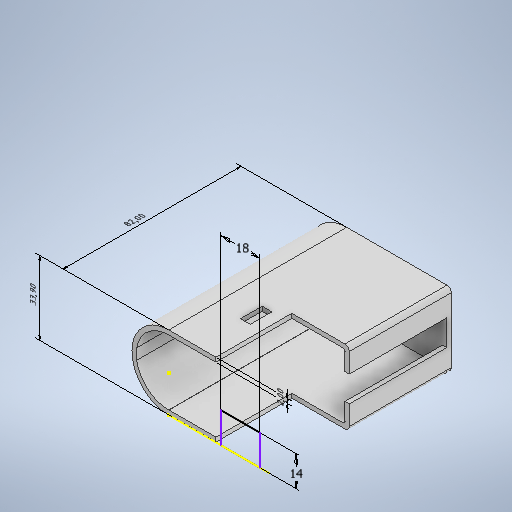
# Autodesk Inventor part: schranka
Saved by Autodesk Inventor 2025.3 (Build 293356000, 356)
## iProperties
Created: 2025-06-12
Part Number: schranka
Material: Generic
Document SubType Name: Modeling
Designer: Repete
Density: 1 g/cm^3
Appearance: Default
Author: Repete
Autodesk Inventor part; units mm, degrees
ref_plane "YZ Plane" through (0, 0, 0) normal (1, 0, 0) x (0, 1, 0)
ref_plane "XZ Plane" through (0, 0, 0) normal (0, 1, 0) x (-1, 0, 0)
sketch "Sketch1" plane through (0, 0, 0) normal (0, 1, 0) x (-1, 0, 0)
  line L0 (-15.6488, -14.9) -> (-4.1777, -14.9)
  line L1 (-4.1777, 15) -> (-13.2013, 15)
  line L2 (14.7902, 2.5) -> (14.8, 2.5)
  line L3 (14.8, 2.5) -> (14.8, -2.5)
  line L4 (14.8, -2.5) -> (14.7902, -2.5)
  arc A0 (0, -15) -> (14.7902, -2.5) centre (0, 0) ccw
  arc A1 (14.7902, 2.5) -> (0, 15) centre (0, 0) ccw
  line L5 (0.0236, 15) -> (0.0236, 15.0064)
  line L6 (0.0236, 15) -> (-4.1777, 15)
  line L7 (-4.1777, 15) -> (-4.1777, 15)
  line L8 (-0.1777, -14.9) -> (-4.1777, -14.9)
  line L9 (-4.1777, -14.9) -> (0, -14.9)
  line L10 (-4.1777, -14.9) -> (-4.1777, -14.9)
  line L11 (-13.2013, 15) -> (-46.2013, 15)
  line L12 (-15.6488, -14.9) -> (-46.2013, -14.9)
  line L13 (-46.2013, -14.9) -> (-46.2013, 15)
  arc A2 (-1.8412, -16.9) -> (0, 17) centre (0, 0) ccw
  line L14 (0, 17) -> (-48.2013, 17)
  line L15 (-48.2013, 17) -> (-48.2013, -16.9)
  line L16 (-48.2013, -16.9) -> (-1.8412, -16.9)
  line L17 (0.0236, 15) -> (0.0236, 15)
  line L18 (0, -14.9) -> (0, -15)
  point P0 (-13.2013, 0)
  point P1 (12.5, 0)
  point P2 (11.0065, 21.7068)
  point P3 (11.0065, 50.7004)
  dimension "d7" = 33
  dimension "d8" = 2
  dimension "d9" = 2
  dimension "d10" = 2
  dimension "d11" = 2
  dimension "d39" = 15
  dimension "d90" = 33.9
  dimension "d91" = 29.9
  dimension "d92" = 2
  dimension "d93" = 2
  dimension "d94" = 2.2
  dimension "d95" = 14.8
  constraints: 38 end point, 7 point on circle, 5 horizontal, 4 parallel, 4 perpendicular, 3 centre point, 1 coincident, 1 vertical
  measures "d7" distance from line of L13 point (-13.201, 0)
  measures "d8" radial gap between concentric circles of A0 A2
  measures "d9" distance between parallel lines of L15 L13
  measures "d10" distance between parallel lines of L0 L16
  measures "d11" distance between parallel lines of L14 L11
  measures "d39" radius of A1
  measures "d90" distance of L14.end L15.end
  measures "d91" distance of L12.end L11.end
  measures "d92" distance between parallel lines of L14 L6
  measures "d93" distance between parallel lines of L16 L8
  measures "d94" distance edge to line of A2 L3
  measures "d95" distance from line of A0.centre L3
extrude "Extrusion1" add sketch "Sketch1" along normal blind 80
ref_plane "Work Plane1" through (0, 82, 0) normal (0, 1, 0) x (1, 0, 0)
sketch "Sketch3" plane through (0, 82, 0) normal (0, 1, 0) x (1, 0, 0)
  arc A0 (0, 17) -> (0, -17) centre (0, 0) ccw
  line L0 (0, -17) -> (48.2013, -17)
  line L1 (48.2013, -17) -> (48.2013, 17)
  line L2 (48.2013, 17) -> (0, 17)
  point P0 (13.2013, 0)
  point P1 (-14.9845, -166.3883)
  point P2 (-14.9845, -137.3947)
  point P3 (-26.1687, -202.0885)
  constraints: 6 end point, 2 point on circle, 1 centre point, 1 parallel, 1 perpendicular
extrude "Extrusion2" add sketch "Sketch3" against normal up to surface (2 mm away)
sketch "Sketch4" plane through (48.2013, 0, -16.9) normal (0, 0, -1) x (-1, 0, 0)
  point P0 (48.2013, 0)
fillet "Fillet1" radius 2 2 edges at (48.2013, 40, -16.9) (48.2013, 41, 17)
fillet "Fillet2" radius 1 2 edges at (46.2013, 40, 15) (46.2013, 40, -14.9)
fillet "Fillet3" radius 2 1 edges at (48.2013, 81, -17)
sketch "Sketch10" plane through (0, 0, 0) normal (0, -1, 0) x (1, 0, 0)
  line L0 (0, -17) -> (46.2013, -17) projected
  line L1 (23.9488, -17) -> (41.9488, -17)
  line L2 (41.9488, -17) -> (41.9488, -3)
  line L3 (41.9488, -3) -> (23.9488, -3)
  line L4 (23.9488, -3) -> (23.9488, -17)
  point P0 (0, 0)
  dimension "d79" = 14
  dimension "d80" = 18
  constraints: 8 end point, 2 parallel, 1 horizontal, 1 perpendicular, 1 point on line
  measures "d79" distance of L1.end L2.end
  measures "d80" distance of L2.end L3.end
sketch "Sketch11" plane through (0, 0, 0) normal (0, -1, 0) x (1, 0, 0)
  line L0 (0, 17) -> (46.2013, 17) projected
  line L1 (21.7013, 17) -> (48.2013, 17)
  line L2 (48.2013, 17) -> (48.2013, -16.9)
  line L3 (48.2013, -16.9) -> (21.7013, -16.9)
  line L4 (21.7013, -16.9) -> (21.7013, 17)
  line L5 (48.2013, 15) -> (48.2013, -14.9) projected
  point P0 (0, 0)
  dimension "d86" = 26.5
  dimension "d87" = 0
  constraints: 8 end point, 2 parallel, 1 horizontal, 1 perpendicular, 1 point on line
  measures "d86" distance between parallel lines of L2 L4
  measures "d87" distance between parallel lines of L5 L2
extrude "Extrusion8" cut sketch "Sketch11" against normal blind 35
sketch "Sketch12" plane through (48.2013, 82, 15) normal (1, 0, 0) x (0, 0, -1)
  line L0 (0, -47) -> (29.9, -47) projected
  line L1 (9, -47) -> (20.9, -47)
  line L2 (20.9, -47) -> (20.9, -2)
  line L3 (20.9, -2) -> (9, -2)
  line L4 (9, -2) -> (9, -47)
  line L5 (29.9, -2) -> (29.9, -47) projected
  line L6 (0, -47) -> (0, 0) projected
  line L7 (0, 0) -> (30, 0) projected
  point P0 (15, -82)
  dimension "d97" = 9
  dimension "d98" = 9
  dimension "d99" = 2
  constraints: 8 end point, 2 parallel, 1 horizontal, 1 perpendicular, 1 point on line
  measures "d97" distance between parallel lines of L5 L2
  measures "d98" distance between parallel lines of L6 L4
  measures "d99" distance between parallel lines of L7 L3
extrude "Extrusion9" cut sketch "Sketch12" against normal up to surface (2 mm away)
sketch "Sketch13" plane through (0, 0, 17) normal (0, 0, 1) x (1, 0, 0)
  line L0 (16.5, 31) -> (12, 31)
  line L1 (12, 31) -> (12, 21)
  line L2 (12, 21) -> (16.5, 21)
  line L3 (16.5, 21) -> (16.5, 31)
  line L4 (0, 0) -> (21.7013, 0) projected
  line L5 (0, 0) -> (0, 82) projected
  line L6 (0, 82) -> (46.2013, 82) projected
  dimension "d103" = 12
  dimension "d107" = 61
  dimension "d108" = 4.5
  dimension "d109" = 10
  constraints: 8 end point, 2 parallel, 1 horizontal, 1 perpendicular
  measures "d103" distance between parallel lines of L5 L1
  measures "d107" distance between parallel lines of L6 L2
  measures "d108" distance between parallel lines of L3 L1
  measures "d109" distance between parallel lines of L2 L0
extrude "Extrusion10" cut sketch "Sketch13" against normal up to surface (2 mm away)
body "Solid1"
